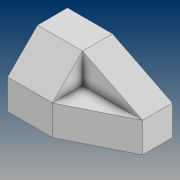
# Autodesk Inventor part: 13-1
Saved by Autodesk Inventor 2020.2 (Build 242310000, 310)
## iProperties
Created: 2020-09-17
Part Number: 13-1
Material: 一般
Document SubType Name: Modeling
Designer: user
Density: 1 g/cm^3
Appearance: 預設
Author: user
Autodesk Inventor part; units mm, degrees
ref_plane "YZ Plane" through (0, 0, 0) normal (1, 0, 0) x (0, 1, 0)
ref_plane "XZ Plane" through (0, 0, 0) normal (0, 1, 0) x (-1, 0, 0)
ref_plane "XY Plane" through (0, 0, 0) normal (0, 0, 1) x (1, 0, 0)
sketch "草圖1" plane through (0, 0, 0) normal (0, 1, 0) x (-1, 0, 0)
  line L0 (0, 0) -> (-70, 0)
  line L1 (-70, 0) -> (-70, -40)
  line L2 (-70, -40) -> (0, -40)
  line L3 (0, -40) -> (0, 0)
  line L4 (-30, 0) -> (-70, -20)
  dimension "d0" = 70
  dimension "d1" = 40
  dimension "d2" = 20
  dimension "d3" = 30
  constraints: 10 end point, 2 parallel, 1 horizontal, 1 midpoint, 1 perpendicular, 1 point on line
  measures "d0" distance of L0.start L0.end
  measures "d1" distance of L2.end L0.start
  measures "d2" distance from line of L2 L4.end
  measures "d3" distance from line of L3 L4.start
extrude "擠出1" add sketch "草圖1" along normal blind 40
sketch "草圖10" plane through (0, 40, 0) normal (0, 1, 0) x (1, 0, 0)
  line L0 (70, 40) -> (70, 0) projected
  line L1 (70, 0) -> (0, 0) projected
  line L2 (0, 0) -> (0, 40) projected
  line L3 (0, 40) -> (70, 40) projected
  line L4 (0, 0) -> (70, 0) projected
  line L5 (70, 0) -> (30, 0)
  line L6 (30, 0) -> (30, 20)
  line L7 (30, 20) -> (70, 20)
  line L8 (70, 20) -> (70, 0)
  point P0 (30, 0)
  dimension "d13" = 30
  dimension "d14" = 20
  constraints: 8 end point, 2 parallel, 1 horizontal, 1 perpendicular
  measures "d13" distance between parallel lines of L6 L2
  measures "d14" distance between parallel lines of L3 L7
extrude "擠出3" cut sketch "草圖10" against normal blind 20 contours L0 L1 L6 L7
sketch "草圖11" plane through (30, 40, 0) normal (1, 0, 0) x (0, 0, -1)
  line L0 (20, -20) -> (20, 0) projected
  line L1 (0, 0) -> (20, 0) projected
  line L2 (0, -20) -> (0, 0) projected
  line L3 (40, -40) -> (0, -40) projected
  line L4 (40, 0) -> (40, -40) projected
  line L5 (20, 0) -> (40, 0) projected
  line L6 (20, 0) -> (0, -20)
  line L7 (0, -40) -> (0, 0) projected
  line L8 (0, -40) -> (0, -20) projected
  line L9 (0, -20) -> (20, -20) projected
  point P0 (0, -20)
  constraints: 2 end point, 1 midpoint
extrude "擠出4" cut sketch "草圖11" against normal through all contours L6 L2 L1
sketch "草圖12" plane through (30, 0, -20) normal (0, 0, 1) x (1, 0, 0)
  line L0 (-30, 40) -> (0, 40) projected
  line L1 (0, 40) -> (40, 40) projected
  line L2 (40, 40) -> (40, 20) projected
  line L3 (40, 0) -> (-30, 0) projected
  line L4 (-30, 0) -> (-30, 40) projected
  line L5 (0, 40) -> (0, 20) projected
  line L6 (0, 40) -> (40, 20)
  line L7 (40, 0) -> (40, 40) projected
  line L8 (40, 20) -> (40, 0) projected
  line L9 (0, 20) -> (40, 20) projected
  constraints: 2 end point, 1 midpoint
extrude "擠出5" cut sketch "草圖12" against normal through all contours L1 L2 L6
sketch "草圖13" plane through (0, 20, 0) normal (0, 1, 0) x (1, 0, 0)
  line L0 (30, 0) -> (0, 0) projected
  line L1 (0, 0) -> (0, 40) projected
  line L2 (0, 40) -> (70, 40) projected
  line L3 (70, 40) -> (70, 20) projected
  line L4 (70, 20) -> (30, 20) projected
  line L5 (30, 20) -> (30, 0) projected
  line L6 (70, 0) -> (30, 0) projected
  line L7 (70, 20) -> (70, 0) projected
  line L8 (70, 20) -> (70, 0) projected
  line L9 (30, 0) -> (70, 20)
  constraints: 2 end point
extrude "擠出6" cut sketch "草圖13" against normal through all contours L9 L7 L6
